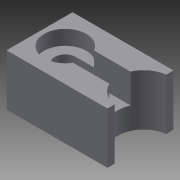
# Autodesk Inventor part: 7.2 Part 2
Saved by Autodesk Inventor 2015 (Build 190159000, 159)
## iProperties
Created: 2015-03-16
Part Number: 7.2 Part 2
Material: Generic
Document SubType Name: Modeling
Designer: PLTW-Stu-02
Density: 1 g/cm^3
Appearance: Default
Author: PLTW-Stu-02
Autodesk Inventor part; units mm, degrees
ref_plane "YZ Plane" through (0, 0, 0) normal (1, 0, 0) x (0, 1, 0)
ref_plane "XZ Plane" through (0, 0, 0) normal (0, 1, 0) x (-1, 0, 0)
ref_plane "XY Plane" through (0, 0, 0) normal (0, 0, 1) x (1, 0, 0)
sketch "Sketch1" plane through (0, 0, 0) normal (0, 1, 0) x (-1, 0, 0)
  line L0 (-110.556, -67.8158) -> (-459.806, -67.8158)
  line L1 (-459.806, -67.8158) -> (-459.806, -296.4158)
  line L2 (-459.806, -296.4158) -> (-110.556, -296.4158)
  line L3 (-110.556, -296.4158) -> (-110.556, -67.8158)
  point P0 (0, 0)
  dimension "d0" = 349.25
  dimension "d1" = 228.6
  constraints: 8 end point, 2 parallel, 1 horizontal, 1 perpendicular
  measures "d0" distance of L2.end L1.end
  measures "d1" distance of L1.end L0.end
extrude "Extrusion2" add sketch "Sketch1" along normal blind 177.8
sketch "Sketch2" plane through (0, 177.8, 0) normal (0, 1, 0) x (1, 0, 0)
  arc A0 (459.806, 271.0158) -> (459.806, 93.2158) centre (470.8722, 182.1158) ccw
  line L0 (459.806, 271.0158) -> (459.806, 93.2158)
  line L1 (459.806, 67.8158) -> (459.806, 296.4158) projected
  point P0 (0, 0)
  constraints: 2 end point, 2 point on circle, 1 centre point, 1 collinear
extrude "Extrusion3" cut sketch "Sketch2" against normal through all
sketch "Sketch3" plane through (0, 177.8, 0) normal (0, 1, 0) x (1, 0, 0)
  line L0 (110.556, 296.4158) -> (110.556, 67.8158) projected
  line L1 (459.806, 296.4158) -> (110.556, 296.4158) projected
  point P0 (0, 0)
  point P1 (199.456, 182.1158)
hole "Hole3" at (199.456, 177.8, -182.1158) direction (0, -1, 0) diameter 146.05 depth 50.8
sketch "Sketch4" plane through (199.456, 127, -182.1158) normal (0, 1, 0) x (1, 0, 0)
  point P0 (-199.456, -182.1158)
  point P1 (0, 0)
hole "Hole5" at (199.456, 127, -182.1158) direction (0, -1, 0) diameter 73.025 end through all
sketch "Sketch5" plane through (0, 177.8, 0) normal (0, 1, 0) x (1, 0, 0)
  circle A0 centre (199.456, 182.1158) radius 36.5125 projected
  line L0 (199.456, 218.6283) -> (389.0644, 218.6283)
  arc A1 (459.806, 271.0158) -> (459.806, 93.2158) centre (470.8722, 182.1158) ccw projected
  line L1 (199.456, 145.6033) -> (389.0644, 145.6033)
  arc A2 (199.456, 145.6033) -> (199.456, 218.6283) centre (199.456, 182.1158) ccw
  arc A3 (389.0644, 218.6283) -> (389.0644, 145.6033) centre (470.8722, 182.1158) ccw
  point P0 (0, 0)
  constraints: 8 point on circle, 4 end point, 4 tangent, 2 centre point, 1 concentric, 1 horizontal, 1 parallel
extrude "Extrusion5" cut sketch "Sketch5" against normal blind 101.6 contours A0 L0 A1 L1
body "Solid2"
